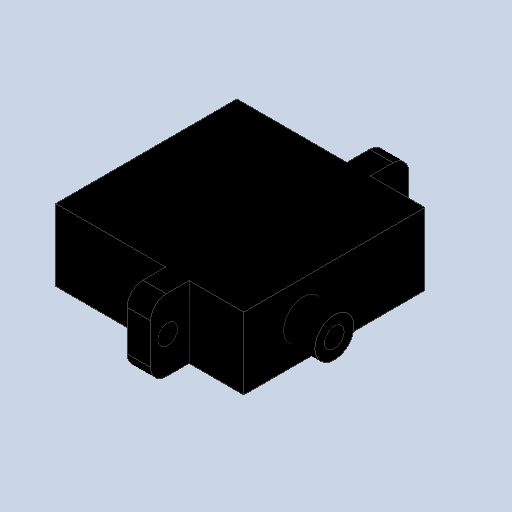
# Autodesk Inventor part: EMAX ES3352 sim
Saved by Autodesk Inventor 2025.2 (Build 292293000, 293)
## iProperties
Category: <PART CATAGORY>
Created: 2025-01-13
Part Number: EMAX ES3352 sim
Material: Generic
Document SubType Name: Modeling
Designer: lachl
Density: 1 g/cm^3
Appearance: Default
Title: <TITLE>
Author: lachl
Revision Number: 1
Autodesk Inventor part; units mm, degrees
ref_plane "YZ Plane" through (0, 0, 0) normal (1, 0, 0) x (0, 1, 0)
ref_plane "XZ Plane" through (0, 0, 0) normal (0, 1, 0) x (-1, 0, 0)
ref_plane "XY Plane" through (0, 0, 0) normal (0, 0, 1) x (1, 0, 0)
sketch "Sketch7" plane through (0, 0, 0) normal (1, 0, 0) x (0, 1, 0)
  line L0 (4.585, 16.5) -> (-4.585, 16.5)
  line L1 (-4.585, 16.5) -> (-4.585, -16.5)
  line L2 (-4.585, -16.5) -> (4.585, -16.5)
  line L3 (4.585, -16.5) -> (4.585, 16.5)
  circle A0 centre (0, 14.3) radius 1.25
  circle A1 centre (0, -14.3) radius 1.25
  line L4 (4.585, 0) -> (-4.585, 0) construction
  line L5 (4.585, 11.585) -> (-4.585, 11.585)
  line L6 (4.585, -11.585) -> (-4.585, -11.585)
  point P0 (0, 0)
  point P1 (0, 16.5)
  point P2 (0, 0)
  dimension "d85" = 33
  dimension "d86" = 9.17
  dimension "d87" = 2.5
  dimension "d89" = 28.6
  dimension "d90" = 23.17
  constraints: 14 end point, 4 midpoint, 4 point on line, 3 perpendicular, 2 centre point, 2 parallel, 2 vertical alignment, 1 equal radius, 1 horizontal, 1 horizontal alignment, 2 other
  measures "d85" distance of L2.end L0.start
  measures "d86" distance of L0.start L0.end
  measures "d87" diameter of A0
  measures "d89" distance of A1.centre A0.centre
  measures "d90" distance between parallel lines of L6 L5
extrude "Extrusion3" add sketch "Sketch7" along normal blind 3
fillet "Fillet1" radius 2 1 edges at (1.5, 4.585, 16.5)
fillet "Fillet2" radius 2 1 edges at (1.5, 4.585, -16.5)
fillet "Fillet3" radius 2 1 edges at (1.5, -4.585, -16.5)
fillet "Fillet4" radius 2 1 edges at (1.5, -4.585, 16.5)
sketch "Sketch8" plane through (3, 0, 0) normal (1, 0, 0) x (0, 0, -1)
  line L0 (14.5, 4.585) -> (-14.5, 4.585) projected
  line L1 (-14.5, -4.585) -> (14.5, -4.585) projected
  line L2 (-11.585, 4.585) -> (11.585, 4.585)
  line L3 (11.585, 4.585) -> (11.585, -4.585)
  line L4 (11.585, -4.585) -> (-11.585, -4.585)
  line L5 (-11.585, -4.585) -> (-11.585, 4.585)
  line L6 (0, 4.585) -> (0, -4.585) construction
  line L7 (-11.585, 4.585) -> (11.585, 4.585)
  line L8 (11.585, -4.585) -> (-11.585, -4.585)
  point P0 (0, 0)
  point P1 (0, 0)
  point P2 (0, 4.585)
  point P3 (-11.585, -4.585)
  point P4 (11.585, 4.585)
  dimension "d97" = 23.17
  constraints: 14 end point, 4 midpoint, 2 collinear, 2 parallel, 2 perpendicular, 2 point on line, 1 horizontal, 1 vertical alignment, 1 other
  measures "d97" distance between parallel lines of L3 L5
extrude "Extrusion4" add sketch "Sketch8" along normal blind 7 and the other way blind 17.05
sketch "Sketch9" plane through (10, 0, 0) normal (1, 0, 0) x (0, 0, -1)
  circle A0 centre (-4, 0) radius 2.5
  point P0 (0, 0)
  dimension "d102" = 5
  dimension "d103" = 4
  constraints: 1 centre point, 1 horizontal alignment
  measures "d102" diameter of A0
  measures "d103" distance of point (0, 0) A0.centre
extrude "Extrusion5" add sketch "Sketch9" along normal blind 4
sketch "Sketch11" plane through (14, 0, 4) normal (1, 0, 0) x (0, 0, -1)
  circle A0 centre (0, 0) radius 1.25
  circle A1 centre (0, 0) radius 2.5 projected
  point P0 (4, 0)
  dimension "d107" = 2.5
  constraints: 1 centre point, 1 concentric
  measures "d107" diameter of A0
extrude "Extrusion6" cut sketch "Sketch11" against normal blind 7 contours A0
body "Solid2"
